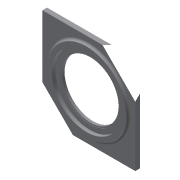
# Autodesk Inventor part: Swerve Pre Baseplate
Saved by Autodesk Inventor 2014 SP1 (Build 180222100, 222)
## iProperties
Created: 2014-05-15
Part Number: Swerve Pre Baseplate
Material: Generic
Document SubType Name: Modeling
Designer: Rauhul Varma
Density: 1 g/cm^3
Appearance: Default
Author: Rauhul Varma
Autodesk Inventor part; units mm, degrees
ref_plane "YZ Plane" through (0, 0, 0) normal (1, 0, 0) x (0, 1, 0)
ref_plane "XZ Plane" through (0, 0, 0) normal (0, 1, 0) x (-1, 0, 0)
ref_plane "XY Plane" through (0, 0, 0) normal (0, 0, 1) x (1, 0, 0)
sketch "Sketch1" plane through (0, 0, 0) normal (0, 0, 1) x (1, 0, 0)
  line L0 (-63.5, -63.5) -> (63.5, -63.5)
  line L1 (63.5, -63.5) -> (63.5, 63.5)
  line L2 (63.5, 63.5) -> (-63.5, 63.5)
  line L3 (-63.5, 63.5) -> (-63.5, -63.5)
  line L4 (-63.5, -63.5) -> (63.5, 63.5) construction
  line L5 (63.5, -63.5) -> (-63.5, 63.5) construction
  circle A0 centre (0, 0) radius 47.5
  circle A1 centre (0, 0) radius 38.77
  circle A2 centre (0, 0) radius 40.635
  dimension "d0" = 127
  dimension "d1" = 127
  dimension "d2" = 95
  dimension "d3" = 77.54
  dimension "d4" = 81.27
  constraints: 12 end point, 3 centre point, 3 coincident, 2 midpoint, 2 parallel, 1 horizontal, 1 perpendicular
  measures "d0" distance of L2.end L1.end
  measures "d1" distance of L1.end L0.end
  measures "d2" diameter of A0
  measures "d3" diameter of A1
  measures "d4" diameter of A2
extrude "Extrusion1" add sketch "Sketch1" against normal blind 9.525 contours L3 L2 L1 L0 | A0 | A2
extrude "Extrusion2" cut sketch "Sketch1" against normal blind 4.7625 contours A0
extrude "Extrusion3" cut sketch "Sketch1" against normal blind 5.1594 contours A2
sketch "Sketch2" plane through (0, 0, -9.525) normal (0, 0, -1) x (-1, 0, 0)
  circle A0 centre (0, 0) radius 38.77 projected
  circle A1 centre (0, 0) radius 38.1
  circle A2 centre (0, 0) radius 48.0219
  dimension "d11" = 76.2
  dimension "d12" = 96.0438
  constraints: 2 centre point, 2 coincident
  measures "d11" diameter of A1
  measures "d12" diameter of A2
extrude "Extrusion4" cut sketch "Sketch2" against normal blind 0.7937 contours A2
sketch "Sketch3" plane through (0, 0, 0) normal (0, 0, 1) x (1, 0, 0)
  line L0 (-63.5, -63.5) -> (63.5, -63.5) projected
  line L1 (63.5, -63.5) -> (63.5, 63.5) projected
  line L2 (63.5, 63.5) -> (-63.5, 63.5) projected
  line L3 (-63.5, 63.5) -> (-63.5, -63.5) projected
  circle A0 centre (0, 0) radius 47.5 projected
  circle A1 centre (0, 0) radius 53.975
  dimension "d16" = 107.95
  constraints: 1 centre point, 1 coincident
  measures "d16" diameter of A1
extrude "Extrusion5" cut sketch "Sketch3" against normal blind 3.175 contours L3 L2 L1 L0
fillet "Fillet1" radius 3.175 1 edges at (-53.975, 0, -3.175)
body "Solid1"
